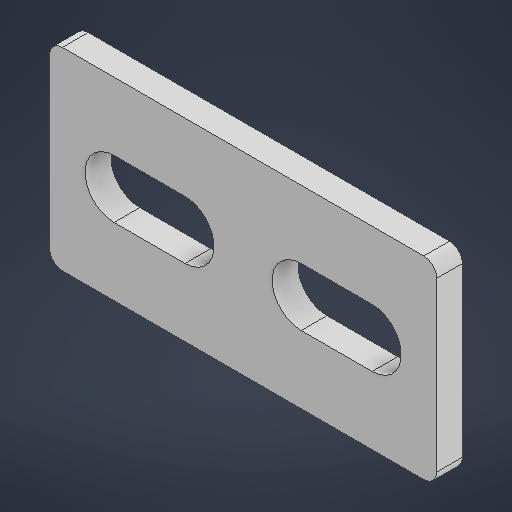
# Autodesk Inventor part: connector_30x30
Saved by Autodesk Inventor 2025.1 (Build 291241000, 241)
## iProperties
Created: 2024-12-20
Part Number: connector_30x30
Material: Všeobecné
Document SubType Name: Modeling
Designer: lukas
Density: 1 g/cm^3
Appearance: Výchozí
Author: lukas
Autodesk Inventor part; units mm, degrees
ref_plane "YZ Plane" through (0, 0, 0) normal (1, 0, 0) x (0, 1, 0)
ref_plane "XZ Plane" through (0, 0, 0) normal (0, 1, 0) x (-1, 0, 0)
ref_plane "XY Plane" through (0, 0, 0) normal (0, 0, 1) x (1, 0, 0)
sketch "Náčrt1" plane through (0, 0, 0) normal (0, 0, 1) x (1, 0, 0)
  line L0 (-42, 0) -> (42, 0) projected
  line L1 (0, -21) -> (0, 21) projected
  line L2 (30, -15) -> (-30, -15)
  line L3 (-30, -15) -> (-30, 15)
  line L4 (-30, 15) -> (30, 15)
  line L5 (30, 15) -> (30, -15)
  point P0 (0, 0)
  dimension "d0" = 60
  dimension "d1" = 30
  constraints: 8 end point, 2 parallel, 1 horizontal, 1 perpendicular, 2 other
  measures "d0" distance of L3.end L4.end
  measures "d1" distance of L4.end L2.start
extrude "Vysunutí1" add sketch "Náčrt1" along normal blind 4
sketch "Náčrt2" plane through (0, 0, 4) normal (0, 0, 1) x (1, 0, 0)
  line L0 (30, 15) -> (-30, 15) projected
  line L1 (-30, 15) -> (-30, -15) projected
  line L2 (-30, -15) -> (30, -15) projected
  line L3 (30, -15) -> (30, 15) projected
  line L4 (-42, 0) -> (42, 0) projected
  line L5 (0, -21) -> (0, 21) projected
  line L6 (-20, 0) -> (-9, 0) construction
  line L7 (-20, -4.5) -> (-9, -4.5)
  line L8 (-9, 4.5) -> (-20, 4.5)
  arc A0 (-20, 4.5) -> (-20, -4.5) centre (-20, 0) ccw
  arc A1 (-9, -4.5) -> (-9, 4.5) centre (-9, 0) ccw
  point P0 (0, 0)
  point P1 (-14.5, 0)
  dimension "d4" = 9
  dimension "d5" = 11
  dimension "d6" = 10
  constraints: 8 end point, 4 point on circle, 4 tangent, 2 centre point, 2 point on line, 1 midpoint, 1 parallel
  measures "d4" diameter of A1
  measures "d5" distance of L6.start L6.end
  measures "d6" distance from line of L1 L6.start
extrude "Vysunutí2" cut sketch "Náčrt2" against normal through all contours A1 L7 A0 L4 | L4 A0 L8 A1
mirror "Zrcadlit1" about plane through (0, 0, 0) normal (1, 0, 0) of "Vysunutí2"
fillet "Zaoblení1" radius 2 4 edges at (-30, 15, 2) (30, 15, 2) (30, -15, 2) (-30, -15, 2)
